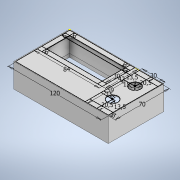
# Autodesk Inventor part: carcassa
Saved by Autodesk Inventor 2022 (Build 260153000, 153)
## iProperties
Created: 2021-05-28
Part Number: carcassa
Material: Generic
Document SubType Name: Modeling
Designer: Pau
Density: 1 g/cm^3
Appearance: Default
Author: Pau
Autodesk Inventor part; units mm, degrees
ref_plane "YZ Plane" through (0, 0, 0) normal (1, 0, 0) x (0, 1, 0)
ref_plane "XZ Plane" through (0, 0, 0) normal (0, 1, 0) x (-1, 0, 0)
ref_plane "XY Plane" through (0, 0, 0) normal (0, 0, 1) x (1, 0, 0)
sketch "Sketch1" plane through (0, 0, 0) normal (0, 1, 0) x (-1, 0, 0)
  line L0 (0, 0) -> (-120, 0)
  line L1 (-120, 0) -> (-120, 70)
  line L2 (-120, 70) -> (0, 70)
  line L3 (0, 70) -> (0, 0)
  dimension "d0" = 120
  dimension "d1" = 70
  constraints: 8 end point, 2 parallel, 1 horizontal, 1 perpendicular
  measures "d0" distance of L1.end L2.end
  measures "d1" distance of L0.end L1.end
extrude "Extrusion1" add sketch "Sketch1" along normal blind 1
sketch "Sketch2" plane through (0, 1, 0) normal (0, 1, 0) x (1, 0, 0)
  line L0 (120, -70) -> (120, 0) projected
  line L1 (120, 0) -> (0, 0) projected
  line L2 (120, -70) -> (90, -70)
  line L3 (90, -70) -> (90, 0)
  line L4 (90, 0) -> (120, 0)
  line L5 (120, 0) -> (120, -70)
  line L6 (0, 0) -> (0, -70) projected
  line L7 (0, -70) -> (90, -70)
  line L8 (90, -70) -> (90, -11)
  line L9 (90, -11) -> (0, -11)
  line L10 (0, -11) -> (0, -70)
  line L11 (0, 0) -> (84, 0)
  line L12 (84, 0) -> (84, -42)
  line L13 (84, -42) -> (0, -42)
  line L14 (0, -42) -> (0, 0)
  line L15 (0, 0) -> (6, 0)
  line L16 (6, 0) -> (6, -6)
  line L17 (6, -6) -> (0, -6)
  line L18 (0, -6) -> (0, 0)
  line L19 (84, 0) -> (78, 0)
  line L20 (78, 0) -> (78, -6)
  line L21 (78, -6) -> (84, -6)
  line L22 (84, -6) -> (84, 0)
  line L23 (90, 0) -> (120, 0)
  line L24 (120, 0) -> (120, -6)
  line L25 (120, -6) -> (90, -6)
  line L26 (90, -6) -> (90, 0)
  line L27 (0, -42) -> (6, -42)
  line L28 (6, -42) -> (6, -36)
  line L29 (6, -36) -> (0, -36)
  line L30 (0, -36) -> (0, -42)
  line L31 (84, -42) -> (78, -42)
  line L32 (78, -42) -> (78, -36)
  line L33 (78, -36) -> (84, -36)
  line L34 (84, -36) -> (84, -42)
  line L35 (90, -70) -> (120, -70)
  line L36 (120, -70) -> (120, -64)
  line L37 (120, -64) -> (90, -64)
  line L38 (90, -64) -> (90, -70)
  line L39 (6, -6) -> (78, -6)
  line L40 (78, -6) -> (78, -36)
  line L41 (78, -36) -> (6, -36)
  line L42 (6, -36) -> (6, -6)
  line L43 (90, 0) -> (105, 0)
  line L44 (105, 0) -> (105, -20.5)
  line L45 (105, -20.5) -> (90, -20.5)
  line L46 (90, -20.5) -> (90, 0)
  circle A0 centre (105, -20.5) radius 6.75
  line L47 (90, -70) -> (105, -70)
  line L48 (105, -70) -> (105, -49.5)
  line L49 (105, -49.5) -> (90, -49.5)
  line L50 (90, -49.5) -> (90, -70)
  circle A1 centre (105, -49.5) radius 6.75
  point P0 (90, -64)
  point P1 (90, -6)
  point P2 (120, -6)
  point P3 (78, 0)
  point P4 (0, -36)
  point P5 (0, -42)
  point P6 (6, -11)
  point P7 (6, -36)
  point P8 (79, -29)
  point P9 (78, -11)
  dimension "d4" = 30
  dimension "d5" = 59
  dimension "d6" = 84
  dimension "d7" = 42
  dimension "d8" = 6
  dimension "d9" = 6
  dimension "d10" = 6
  dimension "d11" = 6
  dimension "d12" = 6
  dimension "d13" = 6
  dimension "d14" = 30
  dimension "d15" = 15
  dimension "d16" = 20.5
  dimension "d17" = 13.5
  dimension "d18" = 15
  dimension "d19" = 20.5
  dimension "d20" = 13.5
  constraints: 96 end point, 24 parallel, 12 horizontal, 12 perpendicular, 9 point on line, 2 centre point, 2 coincident
  measures "d4" distance of L3.end L4.end
  measures "d5" distance of L8.end L7.end
  measures "d6" distance of L12.end L13.end
  measures "d7" distance of L11.end L12.end
  measures "d8" distance of L16.end L17.end
  measures "d9" distance of L15.end L16.end
  measures "d10" distance of L21.end L20.end
  measures "d11" distance of L20.end L19.end
  measures "d12" distance of L28.end L27.end
  measures "d13" distance of L36.end L35.end
  measures "d14" distance of L39.end L40.end
  measures "d15" distance of L44.end L45.end
  measures "d16" distance of L43.end L44.end
  measures "d17" diameter of A0
  measures "d18" distance of L49.end L48.end
  measures "d19" distance of L48.end L47.end
  measures "d20" diameter of A1
extrude "Extrusion2" cut sketch "Sketch2" against normal blind 1 contours A1 L49 L48 | L48 L49 A1 | A0 L45 L44 | L44 L45 A0
extrude "Extrusion3" add sketch "Sketch2" against normal blind 4 contours L2 L48 L37 L0 | L2 L3 L37 L48 | L25 L44 L1 L0 | L25 L3 L1 L44 | L6 L29 L28 L13 | L12 L21 L20 L1 | L32 L33 L12 L13 | L6 L1 L16 L17
extrude "Extrusion4" cut sketch "Sketch2" against normal blind 4 contours L42 L9 L40 L41 | L9 L42 L39 L40
sketch "Sketch5" plane through (0, 1, 0) normal (0, 1, 0) x (1, 0, 0)
  line L0 (0, 0) -> (0, -70) projected
  line L1 (0, 0) -> (-1, 0)
  line L2 (-1, 0) -> (-1, 1)
  line L3 (-1, 1) -> (0, 1)
  line L4 (0, 1) -> (0, 0)
  line L5 (0, -70) -> (-1, -70)
  line L6 (-1, -70) -> (-1, -71)
  line L7 (-1, -71) -> (0, -71)
  line L8 (0, -71) -> (0, -70)
  line L9 (0, -70) -> (120, -70) projected
  line L10 (120, -70) -> (121, -70)
  line L11 (121, -70) -> (121, -71)
  line L12 (121, -71) -> (120, -71)
  line L13 (120, -71) -> (120, -70)
  line L14 (120, -70) -> (120, 0) projected
  line L15 (120, 0) -> (121, 0)
  line L16 (121, 0) -> (121, 1)
  line L17 (121, 1) -> (120, 1)
  line L18 (120, 1) -> (120, 0)
  line L19 (120, 0) -> (0, 0) projected
  line L20 (120, 1) -> (0, 1)
  line L21 (0, 1) -> (0, 0)
  line L22 (0, 0) -> (120, 0)
  line L23 (120, 0) -> (120, 1)
  line L24 (-1, 0) -> (0, 0)
  line L25 (0, 0) -> (0, -70)
  line L26 (0, -70) -> (-1, -70)
  line L27 (-1, -70) -> (-1, 0)
  line L28 (0, -71) -> (120, -71)
  line L29 (120, -71) -> (120, -70)
  line L30 (120, -70) -> (0, -70)
  line L31 (0, -70) -> (0, -71)
  line L32 (121, -70) -> (120, -70)
  line L33 (120, -70) -> (120, 0)
  line L34 (120, 0) -> (121, 0)
  line L35 (121, 0) -> (121, -70)
  dimension "d36" = 1
  dimension "d37" = 1
  dimension "d38" = 1
  dimension "d39" = 1
  dimension "d40" = 1
  dimension "d41" = 1
  dimension "d42" = 1
  dimension "d43" = 1
  constraints: 64 end point, 16 parallel, 8 horizontal, 8 perpendicular
  measures "d36" distance of L2.end L3.end
  measures "d37" distance of L1.end L2.end
  measures "d38" distance of L7.end L6.end
  measures "d39" distance of L6.end L5.end
  measures "d40" distance of L11.end L12.end
  measures "d41" distance of L10.end L11.end
  measures "d42" distance of L17.end L16.end
  measures "d43" distance of L16.end L15.end
extrude "Extrusion5" add sketch "Sketch5" against normal blind 26 contours L0 L5 L27 L1 | L1 L2 L3 L4 | L4 L20 L18 L19 | L8 L7 L6 L5 | L9 L13 L28 L8 | L15 L35 L10 L14 | L18 L17 L16 L15 | L10 L11 L12 L13
sketch "Sketch6" plane through (0, -25, 0) normal (0, -1, 0) x (1, 0, 0)
  line L0 (121, 71) -> (-1, 71) projected
  line L1 (0, 70) -> (120, 70) projected
  line L2 (121, 71) -> (120, 70)
  line L3 (120, 0) -> (0, 0) projected
  line L4 (0, 0) -> (-1, -1)
  line L5 (-0.5, -0.5) -> (120.5, -0.5)
  line L6 (120.5, -0.5) -> (120.5, 70.5)
  line L7 (120.5, 70.5) -> (-0.5, 70.5)
  line L8 (-0.5, 70.5) -> (-0.5, -0.5)
  line L9 (121, -1) -> (-1, -1) projected
  line L10 (121, 71) -> (-1, 71)
  line L11 (-1, 71) -> (-1, -1)
  line L12 (-1, -1) -> (121, -1)
  line L13 (121, -1) -> (121, 71)
  point P0 (121, -1)
  constraints: 20 end point, 4 parallel, 2 horizontal, 2 midpoint, 2 perpendicular
sketch "Sketch7" plane through (0, 1, 0) normal (0, 1, 0) x (1, 0, 0)
  point P0 (0, 0)
extrude "Extrusion6" add sketch "Sketch6" along normal blind 5 contours L2 L7 L8 L4 L11 L0 | L13 L9 L4 L5 L6 L2
body "Solid1"
